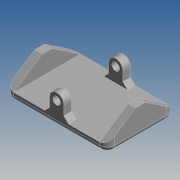
# Autodesk Inventor part: support_pi
Saved by Autodesk Inventor 2017 (Build 210142000, 142)
## iProperties
Created: 2018-10-05
Part Number: support_pi
Material: Générique
Document SubType Name: Modeling
Designer: Gilles Mottiez
Density: 1 g/cm^3
Appearance: Par défaut
Author: Gilles Mottiez
Autodesk Inventor part; units mm, degrees
ref_plane "YZ Plane" through (0, 0, 0) normal (1, 0, 0) x (0, 1, 0)
ref_plane "XZ Plane" through (0, 0, 0) normal (0, 1, 0) x (-1, 0, 0)
ref_plane "XY Plane" through (0, 0, 0) normal (0, 0, 1) x (1, 0, 0)
sketch "Sketch1" plane through (0, 0, 0) normal (0, 0, 1) x (1, 0, 0)
  line L0 (0, 0) -> (90, 0)
  line L1 (90, 0) -> (90, -70)
  line L2 (90, -70) -> (0, -70)
  line L3 (0, -70) -> (0, 0)
  dimension "d0" = 90
  dimension "d1" = 70
  constraints: 8 end point, 2 parallel, 1 horizontal, 1 perpendicular
  measures "d0" distance of L1.end L2.end
  measures "d1" distance of L0.end L1.end
extrude "Extrusion1" add sketch "Sketch1" along normal blind 8
sketch "Esquisse2" plane through (90, -70, 0) normal (1, 0, 0) x (0, 0, -1)
  line L0 (0, 70) -> (0, 0) construction
  line L1 (0, 70) -> (-8, 70) construction
  line L2 (-8, 0) -> (-8, 70) construction
  line L3 (0, 0) -> (-8, 0) construction
  line L4 (-8, 0) -> (-28, 30)
  line L5 (-28, 30) -> (-28, 40)
  line L6 (-28, 40) -> (-8, 70)
  line L7 (0, 35) -> (-8, 35) construction
  line L8 (-8, 0) -> (0, 0)
  line L9 (0, 0) -> (0, 70)
  line L10 (0, 70) -> (-8, 70)
  point P0 (0, 70)
  dimension "d4" = 10
  dimension "d5" = 20
  constraints: 14 end point, 3 collinear, 2 midpoint, 1 vertical, 1 other
  measures "d4" distance of L4.end L5.end
  measures "d5" distance between parallel lines of L2 L5
extrude "Extrusion2" add sketch "Esquisse2" along normal blind 8
sketch "Esquisse3" plane through (0, -70, 0) normal (-1, 0, 0) x (0, 0, 1)
  line L0 (0, 0) -> (0, 70) construction
  line L1 (0, 0) -> (8, 0) construction
  line L2 (8, 70) -> (8, 0) construction
  line L3 (0, 70) -> (8, 70) construction
  line L4 (8, 0) -> (8, 70) construction
  line L5 (8, 0) -> (28, 30) construction
  line L6 (28, 30) -> (28, 40) construction
  line L7 (28, 40) -> (8, 70) construction
  line L8 (8, 70) -> (28, 40)
  line L9 (28, 40) -> (28, 30)
  line L10 (28, 30) -> (8, 0)
  line L11 (8, 0) -> (0, 0)
  line L12 (0, 0) -> (0, 70)
  line L13 (0, 70) -> (8, 70)
  line L14 (0, 35) -> (8, 35) construction
  dimension "d8" = 10
  dimension "d9" = 20
  constraints: 14 end point, 2 midpoint, 2 perpendicular, 1 collinear, 1 vertical, 1 other
  measures "d8" distance of L8.end L9.end
  measures "d9" distance between parallel lines of L2 L9
extrude "Extrusion3" add sketch "Esquisse3" along normal blind 8
sketch "Esquisse4" plane through (90, 0, 8) normal (0, 1, 0) x (1, 0, 0)
  line L0 (-98, 8) -> (8, 8) construction
  line L1 (-98, 0) -> (-98, 8) construction
  line L2 (-90, 0) -> (-98, 0) construction
  line L3 (0, 0) -> (-90, 0) construction
  line L4 (0, 0) -> (8, 0) construction
  line L5 (8, 8) -> (8, 0) construction
  line L6 (-37.5, 0) -> (-52.5, 0) construction
  line L7 (-52.5, 0) -> (-52.5, -15) construction
  line L8 (-52.5, -15) -> (-37.5, -15) construction
  line L9 (-37.5, -15) -> (-37.5, 0) construction
  circle A0 centre (-45, -15) radius 7.5 construction
  line L10 (-52.5, 0) -> (-52.5, -15)
  line L11 (-37.5, 0) -> (-37.5, -15)
  line L12 (-37.5, 0) -> (-52.5, 0)
  arc A1 (-52.5, -15) -> (-37.5, -15) centre (-45, -15) ccw
  point P0 (-90, 8)
  point P1 (-45, 0)
  dimension "d12" = 15
  dimension "d13" = 15
  constraints: 14 end point, 3 collinear, 2 midpoint, 2 parallel, 2 point on circle, 2 tangent, 2 vertical, 1 centre point, 1 coincident, 1 horizontal, 1 horizontal alignment, 1 perpendicular, 1 point on line, 1 vertical alignment, 2 other
  measures "d12" distance of L8.end L7.end
  measures "d13" distance of L7.end L6.end
extrude "Extrusion4" add sketch "Esquisse4" against normal blind 8
sketch "Esquisse5" plane through (90, 0, 8) normal (0, 1, 0) x (1, 0, 0)
  line L0 (-98, 8) -> (8, 8) construction
  line L1 (-98, 0) -> (-98, 8) construction
  line L2 (-90, 0) -> (-98, 0) construction
  line L3 (-52.5, 0) -> (-90, 0) construction
  line L4 (-52.5, -15) -> (-52.5, 0) construction
  arc A0 (-52.5, -15) -> (-37.5, -15) centre (-45, -15) ccw construction
  line L5 (-37.5, 0) -> (-37.5, -15) construction
  line L6 (0, 0) -> (-37.5, 0) construction
  line L7 (0, 0) -> (8, 0) construction
  line L8 (8, 8) -> (8, 0) construction
  circle A1 centre (-45, -15) radius 4
  point P0 (-90, 8)
  dimension "d16" = 8
  constraints: 1 centre point, 1 coincident
  measures "d16" diameter of A1
extrude "Extrusion5" cut sketch "Esquisse5" against normal through all
fillet "Congé1" radius 8 1 edges at (-8, -70, 4)
fillet "Congé2" radius 8 3 edges at (-8, 0, 4) (98, 0, 4) (98, -70, 4)
chamfer "Chanfrein1" distance 5 angle 45 1 edges at (52.5, -4, 8)
chamfer "Chanfrein2" distance 5 angle 45 1 edges at (37.5, -4, 8)
fillet "Congé3" radius 5 8 edges at (95.6569, -2.3431, 0) (98, -35, 0) (95.6569, -67.6569, 0) (45, -70, 0) (-5.6569, -67.6569, 0) (-8, -35, 0) (-5.6569, -2.3431, 0) (45, 0, 0)
sketch "Esquisse6" plane through (0, -70, 8) normal (0, -1, 0) x (1, 0, 0)
  line L0 (90, -3) -> (0, -3) construction
  line L1 (90, 0) -> (90, -3) construction
  line L2 (0, 0) -> (90, 0) construction
  line L3 (0, -3) -> (0, 0) construction
  line L4 (37.5, 0) -> (52.5, 0) construction
  line L5 (52.5, 0) -> (52.5, 15) construction
  line L6 (52.5, 15) -> (37.5, 15) construction
  line L7 (37.5, 15) -> (37.5, 0) construction
  circle A0 centre (45, 15) radius 7.5 construction
  line L8 (37.5, 0) -> (37.5, 15)
  line L9 (52.5, 15) -> (52.5, 0)
  line L10 (37.5, 0) -> (52.5, 0)
  arc A1 (52.5, 15) -> (37.5, 15) centre (45, 15) ccw
  point P0 (0, -8)
  point P1 (45, -3)
  dimension "d28" = 15
  dimension "d29" = 15
  constraints: 14 end point, 3 collinear, 2 midpoint, 2 parallel, 2 point on circle, 2 vertical, 1 centre point, 1 coincident, 1 horizontal, 1 horizontal alignment, 1 perpendicular, 1 point on line, 1 vertical alignment, 3 other
  measures "d28" distance of L5.end L6.end
  measures "d29" distance of L4.end L5.end
extrude "Extrusion6" add sketch "Esquisse6" against normal blind 8
chamfer "Chanfrein3" distance 5 angle 45 2 edges at (52.5, -66, 8) (37.5, -66, 8)
sketch "Esquisse7" plane through (0, -70, 5) normal (0, -1, 0) x (1, 0, 0)
  line L0 (90, 0) -> (0, 0) construction
  line L1 (90, 3) -> (90, 0) construction
  line L2 (57.5, 3) -> (90, 3) construction
  line L3 (52.5, 8) -> (57.5, 3) construction
  line L4 (52.5, 18) -> (52.5, 8) construction
  arc A0 (52.5, 18) -> (37.5, 18) centre (45, 18) ccw construction
  line L5 (37.5, 8) -> (37.5, 18) construction
  line L6 (32.5, 3) -> (37.5, 8) construction
  line L7 (0, 3) -> (32.5, 3) construction
  line L8 (0, 0) -> (0, 3) construction
  circle A1 centre (45, 18) radius 4
  point P0 (0, -5)
  dimension "d35" = 8
  constraints: 1 centre point, 1 coincident
  measures "d35" diameter of A1
extrude "Extrusion7" cut sketch "Esquisse7" against normal through all
